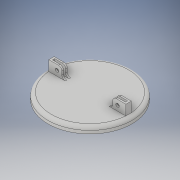
# Autodesk Inventor part: Base
Saved by Autodesk Inventor 2018 (Build 220112000, 112)
## iProperties
Created: 2019-08-28
Part Number: Base
Material: Generic
Document SubType Name: Modeling
Designer: Electro707
Density: 1 g/cm^3
Appearance: Default
Author: Electro707
Autodesk Inventor part; units mm, degrees
ref_plane "YZ Plane" through (0, 0, 0) normal (1, 0, 0) x (0, 1, 0)
ref_plane "XZ Plane" through (0, 0, 0) normal (0, 1, 0) x (-1, 0, 0)
ref_plane "XY Plane" through (0, 0, 0) normal (0, 0, 1) x (1, 0, 0)
sketch "Sketch1" plane through (0, 0, 0) normal (0, 0, 1) x (1, 0, 0)
  line L0 (0, 0) -> (12.065, 0)
  line L1 (71.12, 0) -> (71.12, 9.398)
  line L2 (71.12, 9.398) -> (59.055, 9.398)
  line L3 (0, 9.398) -> (0, 0)
  circle A0 centre (7.62, 4.699) radius 1.6
  circle A1 centre (63.5, 4.699) radius 1.6
  line L4 (63.5, 4.699) -> (7.62, 4.699) construction
  line L5 (12.065, 9.398) -> (12.065, 0)
  line L6 (59.055, 0) -> (59.055, 9.398)
  line L7 (59.055, 9.398) -> (12.065, 9.398) construction
  line L8 (12.065, 9.398) -> (0, 9.398)
  line L9 (12.065, 0) -> (59.055, 0) construction
  line L10 (59.055, 0) -> (71.12, 0)
  line L11 (1.905, 9.398) -> (7.62, 4.699) construction
  line L12 (1.905, 0) -> (7.62, 4.699) construction
  line L13 (63.5, 4.699) -> (69.215, 9.398) construction
  line L14 (69.215, 0) -> (63.5, 4.699) construction
  line L15 (1.905, 0) -> (1.905, 9.398) construction
  line L16 (69.215, 0) -> (69.215, 9.398) construction
  line L17 (1.905, 0) -> (0, 9.398) construction
  line L18 (69.215, 0) -> (71.12, 9.398) construction
  dimension "d0" = 3.2
  dimension "d1" = 55.88
  dimension "d2" = 71.12
  dimension "d3" = 9.398
  dimension "d5" = 67.31
  dimension "d6" = 10.16
  constraints: 38 end point, 11 perpendicular, 10 parallel, 6 point on line, 5 equal length, 4 horizontal, 2 centre point, 1 equal radius
  measures "d0" diameter of A0
  measures "d1" distance of L4.start L4.end
  measures "d2" distance of L1.end L3.start
  measures "d3" distance of L3.start L0.start
  measures "d5" distance between parallel lines of L16 L15
  measures "d6" distance between parallel lines of L15 L5
extrude "Extrusion1" add sketch "Sketch1" along normal blind 5
sketch "Sketch2" plane through (0, 0, 0) normal (0, -1, 0) x (1, 0, 0)
  circle A0 centre (35.56, 2.5) radius 38.735
  line L0 (0, 0) -> (12.065, 0) construction
  line L1 (12.065, 0) -> (12.065, 5) construction
  line L2 (0, 5) -> (12.065, 5) construction
  line L3 (0, 0) -> (0, 5) construction
  line L4 (71.12, 0) -> (59.055, 0) construction
  line L5 (71.12, 0) -> (71.12, 5) construction
  line L6 (59.055, 5) -> (71.12, 5) construction
  line L7 (59.055, 0) -> (59.055, 5) construction
  line L8 (12.065, 5) -> (35.56, 2.5) construction
  line L9 (71.12, 5) -> (59.055, 5) projected
  line L10 (35.56, 2.5) -> (59.055, 5) construction
  line L11 (59.055, 0) -> (71.12, 0) projected
  line L12 (59.055, 0) -> (35.56, 2.5) construction
  dimension "d9" = 77.47
  constraints: 6 end point, 2 equal length, 1 centre point
  measures "d9" diameter of A0
extrude "Extrusion2" add sketch "Sketch2" along normal blind 6
sketch "Sketch3" plane through (0, 9.398, 0) normal (0, 1, 0) x (1, 0, 0)
  line L0 (1.905, -3.5) -> (69.215, -3.5)
  line L1 (69.215, -3.5) -> (69.215, -1.5)
  line L2 (69.215, -1.5) -> (1.905, -1.5)
  line L3 (1.905, -1.5) -> (1.905, -3.5)
  line L4 (71.12, 0) -> (59.055, 0) construction
  line L5 (69.215, -1.5) -> (71.12, 0) construction
  line L6 (71.0194, -5.1196) -> (69.215, -3.5) construction
  line L7 (0, 0) -> (0, -5) construction
  line L8 (0, -5) -> (1.905, -3.5) construction
  line L9 (1.905, -1.5) -> (0, 0) construction
  dimension "d12" = 67.31
  dimension "d13" = 2
  constraints: 16 end point, 3 equal length, 2 parallel, 1 horizontal, 1 perpendicular
  measures "d12" distance of L1.end L2.end
  measures "d13" distance of L2.end L0.start
extrude "Extrusion3" cut sketch "Sketch3" against normal up to surface (9.398 mm away)
fillet "Fillet1" radius 3.175 1 edges at (-3.175, 0, 2.5)
fillet "Fillet2" radius 3.175 8 edges at (12.065, 9.398, 4.25) (12.065, 9.398, 0.75) (12.065, 0, 4.25) (12.065, 0, 0.75) (59.055, 0, 0.75) (59.055, 9.398, 0.75) (59.055, 9.398, 4.25) (59.055, 0, 4.25)
body "Solid1"
